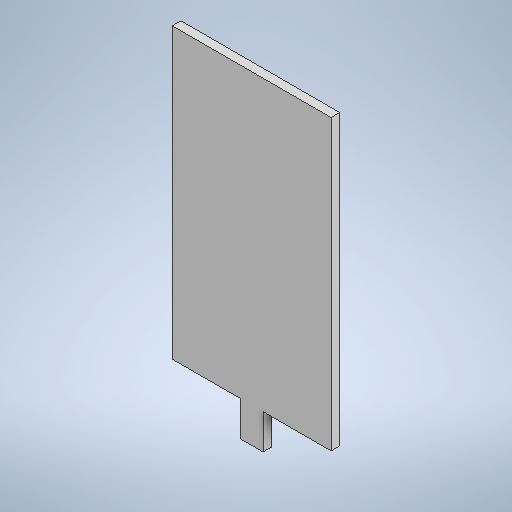
# Autodesk Inventor part: AcrylicPane
Saved by Autodesk Inventor 2025.1 (Build 291241020, 241B)
## iProperties
Created: 2024-09-25
Part Number: AcrylicPane
Material: Generic
Document SubType Name: Modeling
Designer: Si Teng Wu
Density: 1 g/cm^3
Appearance: Default
Author: Si Teng Wu
Autodesk Inventor part; units mm, degrees
ref_plane "YZ Plane" through (0, 0, 0) normal (1, 0, 0) x (0, 1, 0)
ref_plane "XZ Plane" through (0, 0, 0) normal (0, 1, 0) x (-1, 0, 0)
ref_plane "XY Plane" through (0, 0, 0) normal (0, 0, 1) x (1, 0, 0)
sketch "Sketch1" plane through (0, 0, 0) normal (0, 0, 1) x (1, 0, 0)
  line L0 (-27.5, 50) -> (27.5, 50)
  line L1 (27.5, 50) -> (27.5, -50)
  line L2 (27.5, -50) -> (-27.5, -50)
  line L3 (-27.5, -50) -> (-27.5, 50)
  point P0 (0, 0)
  point P1 (0, 50)
  dimension "d0" = 50
  dimension "d2" = 100
  dimension "d3" = 55
  dimension "d4" = 27.5
  constraints: 8 end point, 2 parallel, 1 horizontal, 1 midpoint, 1 perpendicular
  measures "d0" distance of point (0, 50) point (0, 0)
  measures "d2" distance between parallel lines of L2 L0
  measures "d3" distance between parallel lines of L1 L3
  measures "d4" distance from line of L3 point (0, 0)
extrude "Extrusion1" add sketch "Sketch1" along normal blind 3
sketch "Sketch2" plane through (-27.5, -50, 0) normal (0, -1, 0) x (1, 0, 0)
  line L0 (31.45, 0) -> (23.55, 0)
  line L1 (23.55, 0) -> (23.55, 3)
  line L2 (23.55, 3) -> (31.45, 3)
  line L3 (31.45, 3) -> (31.45, 0)
  line L4 (31.45, 0) -> (23.55, 3) construction
  line L5 (23.55, 0) -> (31.45, 3) construction
  line L6 (0, 0) -> (55, 0) projected
  line L7 (0, 3) -> (55, 3) projected
  line L8 (55, 0) -> (55, 3) projected
  line L9 (0, 0) -> (0, 3) projected
  point P0 (27.5, 0)
  point P1 (27.5, 1.5)
  point P2 (55, 1.5)
  point P3 (31.45, 1.5)
  point P4 (0, 1.5)
  point P5 (27.5, 0)
  dimension "d8" = 7.9
  constraints: 12 end point, 6 midpoint, 2 collinear, 2 parallel, 1 horizontal, 1 perpendicular, 1 vertical alignment
  measures "d8" distance between parallel lines of L3 L1
extrude "Extrusion2" add sketch "Sketch2" along normal blind 12.1 contours L0 L1 L2 L3
body "Solid1"
